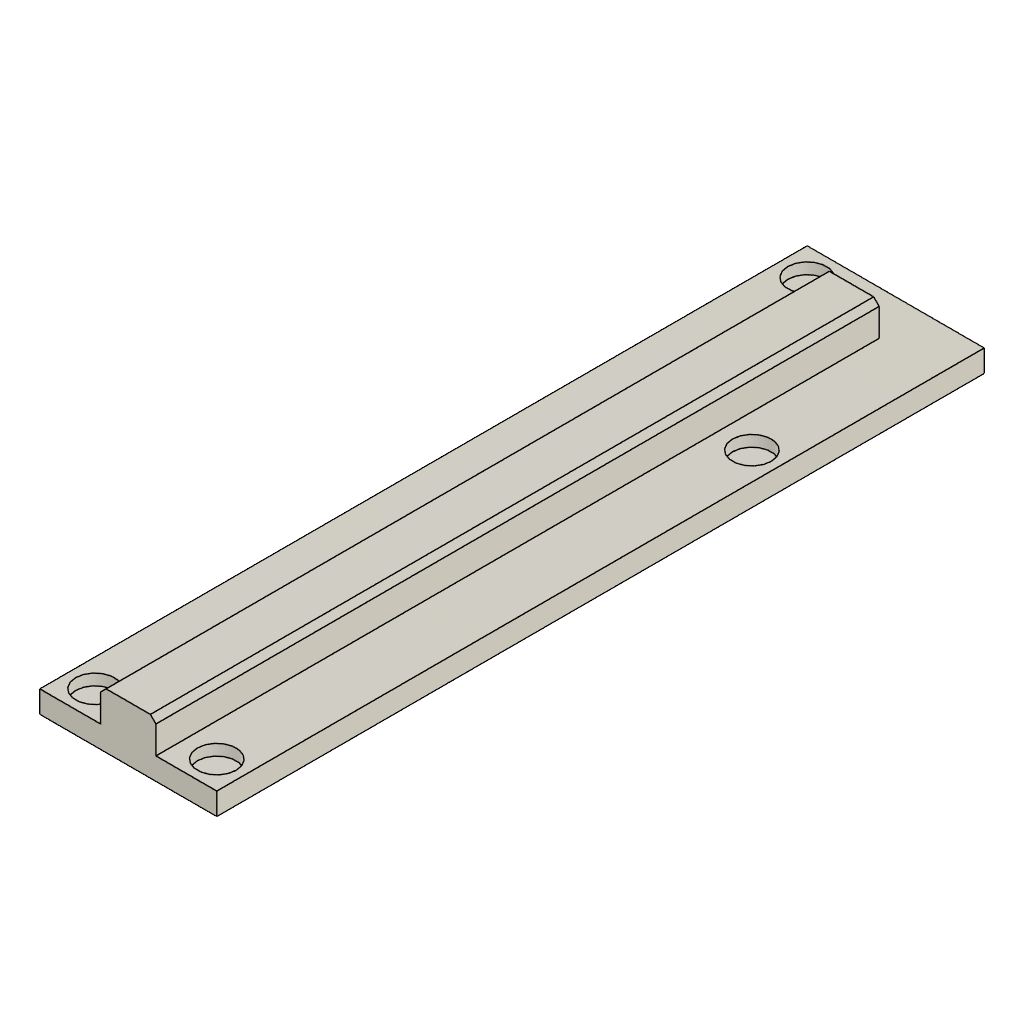
smartie_hopper_mechanism_conduit_1_top (Autodesk Fusion 360 design; units mm, degrees)
part number: 2026-09-19-15-15-46-900
Autodesk Fusion 360 part; units mm, degrees
sketch "3D-printed conduit top outline" plane through (0, 0, 0) normal (0, 1, 0) x (1, 0, 0)
  line L0 (0, 0) -> (16, 0)
  line L1 (16, 0) -> (16, -2)
  line L2 (16, -2) -> (0, -2)
  line L3 (0, -2) -> (0, 0)
  dimension "d7" = 16
  dimension "d8" = 2
  constraint horizontal L0
  constraint vertical L1
  constraint horizontal L2
  constraint vertical L3
  constraint coincident L0.start L3.end
  measures "d7" distance of L0.start L0.end
  measures "d8" distance of L0.start L2.end
extrude "Extrude1" add sketch "3D-printed conduit top outline" along normal blind 69.355
sketch "Magnet holes" plane through (0, 0, 2) normal (0, 0, 1) x (-1, 0, 0)
  line L0 (0, 0) -> (-16, 0)
  line L1 (-16, 0) -> (-16, -69.355)
  line L2 (-16, -69.355) -> (0, -69.355)
  line L3 (0, -69.355) -> (0, 0)
  circle A0 centre (-2.5, -2.5) radius 2.5
  circle A1 centre (-13.5, -2.5) radius 2.5
  circle A2 centre (-2.5, -2.5) radius 1.75
  circle A3 centre (-13.5, -2.5) radius 1.75
  circle A4 centre (-2.5, -66.855) radius 1.75
  circle A5 centre (-2.5, -66.855) radius 2.5
  circle A6 centre (-13.5, -50.855) radius 2.5
  circle A7 centre (-13.5, -50.855) radius 1.75
  dimension "d11" = 5
  dimension "d12" = 5
  dimension "d13" = 3.5
  dimension "d14" = 3.5
  dimension "d17" = 0
  dimension "d18" = -64.355
  dimension "d32" = 0
  dimension "d33" = -48.355
  constraint concentric A0 A2
  constraint concentric A1 A3
  constraint tangent L3 A0
  constraint tangent L0 A0
  constraint tangent L1 A1
  constraint tangent L0 A1
  measures "d11" diameter of A0
  measures "d12" diameter of A1
  measures "d13" diameter of A2
  measures "d14" diameter of A3
extrude "Extrude4" cut sketch "Magnet holes" against normal blind 1 contours A2 | A3 | A4 | A7
sketch "Support rib" plane through (0, 0, 2) normal (0, 0, 1) x (-1, 0, 0)
  circle A0 centre (-13.5, -2.5) radius 1.75
  circle A1 centre (-2.5, -66.855) radius 1.75
  circle A2 centre (-2.5, -2.5) radius 1.75
  circle A3 centre (-13.5, -50.855) radius 1.75
  line L0 (0, 0) -> (-16, 0)
  line L1 (-16, 0) -> (-16, -69.355)
  line L2 (-16, -69.355) -> (0, -69.355)
  line L3 (0, -69.355) -> (0, 0)
  line L4 (-5.5, 0) -> (-10.5, 0)
  line L5 (-10.5, 0) -> (-10.5, -65.355)
  line L6 (-10.5, -65.355) -> (-5.5, -65.355)
  line L7 (-5.5, -65.355) -> (-5.5, 0)
  dimension "d36" = 5
  dimension "d37" = 5.5
  dimension "d38" = 5.5
  dimension "d39" = 4
  constraint horizontal L4
  constraint vertical L5
  constraint horizontal L6
  constraint vertical L7
  constraint coincident L0 L4.start
  measures "d36" distance of L5 L7
  measures "d37" distance of L3 L7
  measures "d38" distance of L1 L5
  measures "d39" distance of L2 L6
extrude "Extrude3" add sketch "Support rib" along normal blind 3 contours L0 L4 L5 L6 L7
chamfer "Chamfer2" distance 0.5 angle 45 2 edges at (10.5, 32.6775, 5) (5.5, 32.6775, 5)
equation "conduit_length = 69.355 mm"
equation "conduit_width = 16 mm"
equation "conduit_wall_thickness = 2 mm"
equation "magnet_diameter = 3 mm"
equation "magnet_height = 1 mm"
equation "number_of_magnets_on_a_side = 2"
equation "d7 = conduit_width"
equation "d8 = conduit_wall_thickness"
equation "d9 = conduit_length"
equation "d11 = magnet_diameter + 2 mm"
equation "d12 = magnet_diameter + 2 mm"
equation "d13 = magnet_diameter + 0.5 mm"
equation "d14 = magnet_diameter + 0.5 mm"
equation "d16 = number_of_magnets_on_a_side"
equation "d18 = -conduit_length + ( magnet_diameter + 2 mm )"
equation "rib_width = 5 mm"
equation "rib_height = 3 mm"
equation "d26 = rib_height"
equation "rib_chamfer = 0.5 mm"
equation "d31 = number_of_magnets_on_a_side"
equation "d33 = -conduit_length + ( magnet_diameter + 2 mm ) + ( conduit_width )"
equation "d34 = -magnet_height"
equation "d36 = rib_width"
equation "d37 = ( conduit_width - rib_width ) / 2"
equation "d39 = 2 * conduit_wall_thickness"
equation "d40 = rib_chamfer"
named bodies: "Smartie hopper mechanism conduit 1 top"
